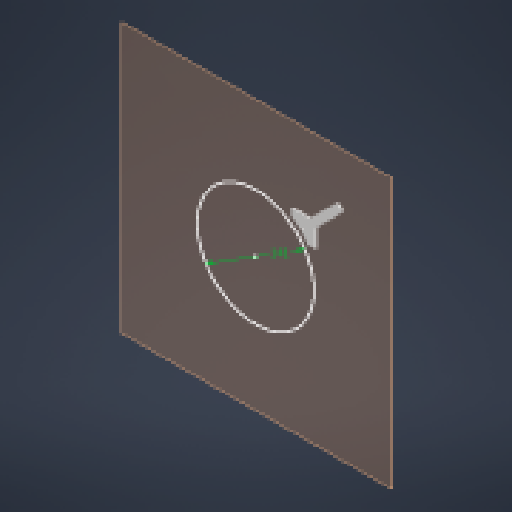
# Autodesk Inventor part: StripMount
Saved by Autodesk Inventor 2023.1 (Build 271208000, 208)
## iProperties
Created: 2023-08-24
Part Number: StripMount
Material: Generic
Document SubType Name: Modeling
Designer: washichi
Density: 1 g/cm^3
Appearance: Default
Author: washichi
Autodesk Inventor part; units mm, degrees
ref_plane "YZ Plane" through (0, 0, 0) normal (1, 0, 0) x (0, 1, 0)
ref_plane "XZ Plane" through (0, 0, 0) normal (0, 1, 0) x (-1, 0, 0)
ref_plane "XY Plane" through (0, 0, 0) normal (0, 0, 1) x (1, 0, 0)
ref_plane "Work Plane1" through (0, 0, 0) normal (0, 0, 1) x (1, 0, 0)
sketch "Sketch1" plane through (0, 0, 0) normal (0, 0, 1) x (1, 0, 0)
  circle A0 centre (0, 0) radius 77.5
  circle A1 centre (0, 0) radius 87.5
  line L0 (0, 0) -> (103.9447, 103.9447)
  line L1 (0, 0) -> (147, 0) construction
  line L2 (103.9447, 96.8736) -> (12.0711, 5)
  line L3 (12.0711, 5) -> (147, 5)
  line L4 (96.8736, 103.9447) -> (-12.0711, -5)
  line L5 (-12.0711, -5) -> (147, -5)
  line L6 (101.1163, 103.9447) -> (103.9447, 101.1163)
  arc A2 (101.1163, 103.9447) -> (96.8736, 103.9447) centre (98.9949, 101.8234) ccw
  arc A3 (103.9447, 96.8736) -> (103.9447, 101.1163) centre (101.8234, 98.9949) ccw
  line L7 (43.5, 72.5) -> (72.5, 72.5)
  line L8 (72.5, 72.5) -> (72.5, 43.5)
  line L9 (72.5, 43.5) -> (43.5, 43.5)
  line L10 (43.5, 43.5) -> (43.5, 72.5)
  line L11 (43.5, 72.5) -> (72.5, 43.5) construction
  line L12 (72.5, 72.5) -> (43.5, 43.5) construction
  circle A4 centre (58, 58) radius 1.5
  point P0 (58.0079, 58.0079)
  point P1 (72.5, 65.4289)
  point P2 (65.4289, 72.5)
  point P3 (43.5, 64.1405)
  point P4 (64.1405, 43.5)
  dimension "d0" = 155
  dimension "d1" = 10
  dimension "d2" = 147
  dimension "d3" = 45
  dimension "d4" = 5
  dimension "d5" = 5
  dimension "d6" = 3
  dimension "d7" = 29
  dimension "d8" = 29
  dimension "d9" = 3
  constraints: 26 end point, 5 centre point, 4 point on circle, 4 tangent, 2 coincident, 2 horizontal, 2 midpoint, 2 parallel, 2 point on line, 1 equal length, 1 equal radius, 1 perpendicular, 2 other
  measures "d0" diameter of A0
  measures "d1" radial gap between concentric circles of A0 A1
  measures "d2" distance of L0.start L0.end
  measures "d3" angle of L1 L0
  measures "d4" distance between parallel lines of L0 L2
  measures "d5" distance between parallel lines of L0 L4
  measures "d6" radius of A2
  measures "d7" distance of L8.end L9.end
  measures "d8" distance of L7.end L8.end
  measures "d9" diameter of A4
extrude "Extrusion2" add sketch "Sketch1" along normal blind 2 contours A0 L2 A1 L8 L9 | L10 L7 A1 L4 A0 | A0 L0 A4 A1 L2 | A1 L2 L8 | L4 A1 L0 A4 A0 | L7 L4 A1 | A1 L0 L8 L2 | L8 L0 L6 A3 L2 | L4 L7 L0 A1 | L4 A2 L6 L0 L7
sketch "Sketch4" plane through (0, 0, 2) normal (0, 0, 1) x (1, 0, 0)
  circle A0 centre (0, 0) radius 70.5
  dimension "d14" = 141
  constraints: 1 centre point, 1 coincident
  measures "d14" diameter of A0
body "Solid2"
